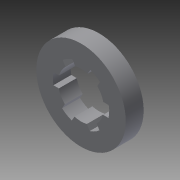
# Autodesk Inventor part: coupler window motor
Saved by Autodesk Inventor 2014 SP1 (Build 180222100, 222)
## iProperties
Created: 2014-01-05
Part Number: coupler window motor
Material: Generic
Document SubType Name: Modeling
Designer: Arpan
Density: 1 g/cm^3
Appearance: Default
Author: Arpan
Autodesk Inventor part; units mm, degrees
ref_plane "YZ Plane" through (0, 0, 0) normal (1, 0, 0) x (0, 1, 0)
ref_plane "XZ Plane" through (0, 0, 0) normal (0, 1, 0) x (-1, 0, 0)
ref_plane "XY Plane" through (0, 0, 0) normal (0, 0, 1) x (1, 0, 0)
sketch "Sketch1" plane through (0, 0, 0) normal (0, 0, 1) x (1, 0, 0)
  circle A0 centre (0, 0) radius 15.875
  line L0 (7.8823, 1.8652) -> (9.8245, 1.8652)
  arc A1 (9.7695, -2.1348) -> (9.8245, 1.8652) centre (0, 0) ccw
  line L1 (9.7695, -2.1348) -> (7.8136, -2.1348)
  arc A2 (5.5564, -5.8937) -> (7.8136, -2.1348) centre (0, 0) ccw
  line L2 (5.5564, -5.8937) -> (6.5275, -7.5757)
  arc A3 (3.0359, -9.528) -> (6.5275, -7.5757) centre (0, 0) ccw
  line L3 (3.0359, -9.528) -> (2.058, -7.8342)
  arc A4 (-2.3259, -7.7589) -> (2.058, -7.8342) centre (0, 0) ccw
  line L4 (-2.3259, -7.7589) -> (-3.297, -9.4409)
  arc A5 (-6.7336, -7.3932) -> (-3.297, -9.4409) centre (0, 0) ccw
  line L5 (-6.7336, -7.3932) -> (-5.7556, -5.6994)
  arc A6 (-7.8823, -1.8652) -> (-5.7556, -5.6994) centre (0, 0) ccw
  line L6 (-7.8823, -1.8652) -> (-9.8245, -1.8652)
  arc A7 (-9.7695, 2.1348) -> (-9.8245, -1.8652) centre (0, 0) ccw
  line L7 (-9.7695, 2.1348) -> (-7.8136, 2.1348)
  arc A8 (-5.5564, 5.8937) -> (-7.8136, 2.1348) centre (0, 0) ccw
  line L8 (-5.5564, 5.8937) -> (-6.5275, 7.5757)
  arc A9 (-3.0359, 9.528) -> (-6.5275, 7.5757) centre (0, 0) ccw
  line L9 (-3.0359, 9.528) -> (-2.058, 7.8342)
  arc A10 (2.3259, 7.7589) -> (-2.058, 7.8342) centre (0, 0) ccw
  line L10 (2.3259, 7.7589) -> (3.297, 9.4409)
  arc A11 (6.7336, 7.3932) -> (3.297, 9.4409) centre (0, 0) ccw
  line L11 (6.7336, 7.3932) -> (5.7556, 5.6994)
  arc A12 (7.8823, 1.8652) -> (5.7556, 5.6994) centre (0, 0) ccw
  constraints: 24 end point, 24 point on circle, 13 centre point
extrude "Extrusion1" add sketch "Sketch1" along normal blind 6.35
body "Solid1"
